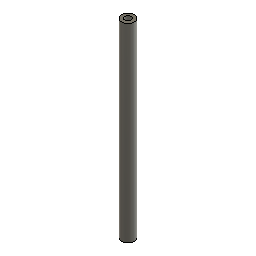
Pole (Autodesk Fusion 360 design; units mm, degrees)
part number: 2026-07-13-22-50-41-633
Autodesk Fusion 360 part; units mm, degrees
sketch "Sketch1" plane through (0, 0, 0) normal (0, 1, 0) x (1, 0, 0)
sketch "Sketch2" plane through (0, 0, 0) normal (0, 1, 0) x (1, 0, 0)
  circle A0 centre (0, 0) radius 5
  dimension "d21" = 10
  constraint coincident A0.centre origin
  measures "d21" diameter of A0
extrude "Extrude3" add sketch "Sketch2" along normal blind 150
hole "Hole6" at (0, 150, 0) direction (0, -1, 0) diameter 5 depth 50 tip angle 180
hole "Hole7" at (0, 0, 0) direction (0, 1, 0) diameter 4.9 depth 4 tip angle 180
